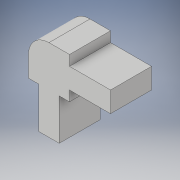
# Autodesk Inventor part: MonsterHolderSupport3
Saved by Autodesk Inventor 2019 (Build 230136000, 136)
## iProperties
Created: 2018-12-05
Part Number: MonsterHolderSupport3
Material: Generic
Document SubType Name: Modeling
Designer: Administrator
Density: 1 g/cm^3
Appearance: Default
Author: Administrator
Autodesk Inventor part; units mm, degrees
ref_plane "YZ Plane" through (0, 0, 0) normal (1, 0, 0) x (0, 1, 0)
ref_plane "XZ Plane" through (0, 0, 0) normal (0, 1, 0) x (-1, 0, 0)
ref_plane "XY Plane" through (0, 0, 0) normal (0, 0, 1) x (1, 0, 0)
sketch "Sketch1" plane through (0, 0, 0) normal (0, 0, 1) x (1, 0, 0)
  line L0 (0, 0) -> (6.35, 0)
  line L1 (6.35, 0) -> (6.35, 6.35)
  line L2 (6.35, 6.35) -> (0, 6.35)
  line L3 (0, 6.35) -> (0, 0)
  dimension "d0" = 6.35
  dimension "d1" = 6.35
  constraints: 8 end point, 2 parallel, 1 horizontal, 1 perpendicular
  measures "d0" distance of L1.end L2.end
  measures "d1" distance of L2.end L0.start
extrude "Extrusion1" add sketch "Sketch1" along normal blind 6.35
sketch "Sketch2" plane through (6.35, 0, 0) normal (1, 0, 0) x (0, 0, -1)
  line L0 (0, 6.35) -> (-6.35, 6.35) projected
  line L1 (-4.7625, 6.35) -> (-1.5875, 6.35)
  line L2 (0, 0) -> (0, 6.35) projected
  line L3 (-6.35, 0) -> (-6.35, 6.35) projected
  line L4 (-6.35, 4.7625) -> (0, 4.7625)
  line L5 (0, 4.7625) -> (0, 1.5875)
  line L6 (0, 1.5875) -> (-6.35, 1.5875)
  line L7 (-6.35, 1.5875) -> (-6.35, 4.7625)
  line L8 (0, 0) -> (-6.35, 0) projected
  dimension "d13" = 3.175
  dimension "d14" = 1.5875
  constraints: 10 end point, 3 point on line, 2 horizontal, 2 parallel, 1 perpendicular
  measures "d13" distance between parallel lines of L4 L6
  measures "d14" distance between parallel lines of L8 L6
sketch "Sketch3" plane through (0, 0, 0) normal (0, -1, 0) x (1, 0, 0)
  line L0 (6.35, 0) -> (0, 0) projected
  line L1 (1.5875, 6.35) -> (4.7625, 6.35)
  line L2 (4.7625, 6.35) -> (4.7625, 0)
  line L3 (4.7625, 0) -> (1.5875, 0)
  line L4 (1.5875, 0) -> (1.5875, 6.35)
  line L5 (6.35, 0) -> (6.35, 6.35) projected
  line L6 (0, 6.35) -> (6.35, 6.35) projected
  line L7 (0, 0) -> (0, 6.35) projected
  point P0 (6.35, 4.7625)
  dimension "d9" = 3.175
  dimension "d10" = 0
  dimension "d17" = 1.5875
  constraints: 8 end point, 2 parallel, 1 horizontal, 1 perpendicular, 1 point on line
  measures "d9" distance between parallel lines of L4 L2
  measures "d10" distance between parallel lines of L6 L1
  measures "d17" distance between parallel lines of L7 L4
extrude "Extrusion3" add sketch "Sketch3" along normal blind 6.35 contours L0 L4 L1 L2
extrude "Extrusion4" add sketch "Sketch2" along normal blind 6.35 contours L2 L6 L3 L4
fillet "Fillet1" radius 3.175 1 edges at (0, 6.35, 3.175)
body "Solid1"
